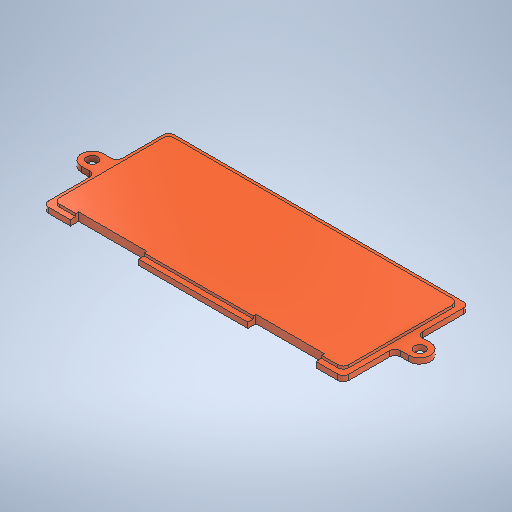
# Autodesk Inventor part: StereoPiBracketLid
Saved by Autodesk Inventor 2025 (Build 290162010, 162A)
## iProperties
Created: 2024-08-20
Part Number: StereoPiBracketLid
Material: Generic
Document SubType Name: Modeling
Designer: 16366081
Density: 1 g/cm^3
Appearance: Default
Author: 16366081
Autodesk Inventor part; units mm, degrees
ref_plane "YZ Plane" through (0, 0, 0) normal (1, 0, 0) x (0, 1, 0)
sketch "Sketch1" plane through (0, 0, 0) normal (0, 1, 0) x (-1, 0, 0)
  line L0 (55, 23) -> (-55, 23)
  line L1 (-55, 23) -> (-55, -23)
  line L2 (-55, -23) -> (55, -23)
  line L3 (55, -23) -> (55, 23)
  line L4 (55, 23) -> (-55, -23) construction
  line L5 (-55, 23) -> (55, -23) construction
  circle A0 centre (60, 0) radius 2
  circle A1 centre (-60, 0) radius 2
  arc A2 (60, -4) -> (60, 4) centre (60, 0) ccw
  line L6 (55, -4) -> (60, -4)
  line L7 (60, 4) -> (55, 4)
  line L8 (55, 4) -> (55, -4)
  arc A3 (-60, 4) -> (-60, -4) centre (-60, 0) ccw
  line L9 (-55, -4) -> (-60, -4)
  line L10 (-60, 4) -> (-55, 4)
  line L11 (-55, 4) -> (-55, -4)
  point P0 (0, 0)
  point P1 (55, 0)
  point P2 (-55, 0)
  point P3 (55, 0)
  point P4 (-55, 0)
  dimension "d0" = 110
  dimension "d1" = 46
  dimension "d2" = 4
  dimension "d3" = 5
  dimension "d4" = 4
  dimension "d5" = 5
  dimension "d6" = 8
  dimension "d7" = 5
  dimension "d8" = 4
  dimension "d9" = 8
  dimension "d10" = 5
  dimension "d11" = 4
  constraints: 24 end point, 6 midpoint, 4 centre point, 4 parallel, 4 point on circle, 3 horizontal, 2 coincident, 2 horizontal alignment, 2 point on line, 2 vertical, 1 perpendicular
  measures "d0" distance of L2.end L1.end
  measures "d1" distance of L1.end L0.end
  measures "d2" diameter of A0
  measures "d3" distance of point (55, 0) A0.centre
  measures "d4" diameter of A1
  measures "d5" distance of point (-55, 0) A1.centre
  measures "d6" diameter of A2
  measures "d7" distance of L6.start L6.end
  measures "d8" distance of point (55, 0) L6.start
  measures "d9" diameter of A3
  measures "d10" distance of L9.start L9.end
  measures "d11" distance of L9.start point (-55, 0)
extrude "Extrusion1" add sketch "Sketch1" along normal blind 2
sketch "Sketch2" plane through (0, 2, 0) normal (0, 1, 0) x (1, 0, 0)
  line L0 (-53, -21) -> (53, -21)
  line L1 (53, -21) -> (53, 21)
  line L2 (53, 21) -> (-53, 21)
  line L3 (-53, 21) -> (-53, -21)
  line L4 (-53, -21) -> (53, 21) construction
  line L5 (53, -21) -> (-53, 21) construction
  point P0 (0, 0)
  dimension "d14" = 106
  dimension "d15" = 42
  constraints: 12 end point, 2 midpoint, 2 parallel, 1 horizontal, 1 perpendicular
  measures "d14" distance of L2.end L1.end
  measures "d15" distance of L1.end L0.end
extrude "Extrusion2" add sketch "Sketch2" along normal blind 1
fillet "Fillet1" radius 2 12 edges at (53, 2.5, 21) (55, 1, 23) (55, 1, 4) (55, 1, -4) (55, 1, -23) (53, 2.5, -21) (-55, 1, -23) (-53, 2.5, -21) (-55, 1, -4) (-55, 1, 4) (-53, 2.5, 21) (-55, 1, 23)
sketch "Sketch3" plane through (0, 0, 0) normal (0, -1, 0) x (1, 0, 0)
  line L0 (-53, 23) -> (53, 23) projected
  line L1 (-45, 23) -> (-20, 23)
  line L2 (-20, 23) -> (-20, 20)
  line L3 (-20, 20) -> (-45, 20)
  line L4 (-45, 20) -> (-45, 23)
  line L5 (20, 23) -> (45, 23)
  line L6 (45, 23) -> (45, 20)
  line L7 (45, 20) -> (20, 20)
  line L8 (20, 20) -> (20, 23)
  line L9 (-55, 6) -> (-55, 21) projected
  line L10 (55, 21) -> (55, 6) projected
  point P0 (0, 0)
  point P1 (-45, 21.5)
  point P2 (45, 21.5)
  dimension "d19" = 25
  dimension "d20" = 3
  dimension "d21" = 25
  dimension "d22" = 3
  dimension "d23" = 10
  dimension "d24" = 10
  constraints: 16 end point, 4 parallel, 2 horizontal, 2 midpoint, 2 perpendicular, 2 point on line
  measures "d19" distance of L2.end L3.end
  measures "d20" distance of L1.end L2.end
  measures "d21" distance of L6.end L7.end
  measures "d22" distance of L5.end L6.end
  measures "d23" distance from line of L9 point (-45, 21.5)
  measures "d24" distance from line of L10 point (45, 21.5)
extrude "Extrusion3" cut sketch "Sketch3" against normal through all
ref_plane "Work Plane1" through (64, 2, 0) normal (0, 0, -1) x (-1, 0, 0)
ref_plane "Work Plane2" through (0, 2, -23) normal (-1, 0, 0) x (0, -1, 0)
body "Solid1"
